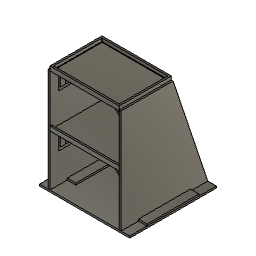
Restaurant Robot Server (v6) (Autodesk Fusion 360 design; units mm, degrees)
Autodesk Fusion 360 part; units mm, degrees
sketch "Sketch1" plane through (0, 0, 0) normal (1, 0, 0) x (0, 1, 0)
  line L0 (0, 0) -> (500, 0)
  line L1 (0, 0) -> (0, 600)
  line L2 (0, 600) -> (300, 600)
  line L3 (300, 600) -> (500, 0)
  dimension "d5" = 600
  constraint coincident L0.start L1.start
  constraint perpendicular L0 L1
  constraint perpendicular L1 L2
  measures "d5" distance of L0.start L1.end
extrude "Extrude1" add sketch "Sketch1" along normal blind 10 makes body 1
move_body "Move1" bodies 1 to x (1, 0, 0) y (0, 1, 0) z (0, 0, 1) at (400, 0, 0)
sketch "Sketch2" plane through (0, 0, 0) normal (1, 0, 0) x (0, 1, 0)
  line L0 (500, 0) -> (0, 0)
  line L1 (0, 0) -> (0, 600)
  line L2 (0, 600) -> (300, 600)
  line L3 (500, 0) -> (300, 600)
  constraint coincident L0.end L1.start
  constraint perpendicular L0 L1
  constraint perpendicular L1 L2
extrude "Extrude2" add sketch "Sketch2" against normal blind 10 separate body makes body 2
move_body "Move2" bodies 2 1 to x (1, 0, 0) y (0, 1, 0) z (0, 0, 1) at (0, 0, 300)
sketch "Sketch3" plane through (0, 0, 300) normal (0, 0, -1) x (1, 0, 0)
  line L0 (0, -500) -> (0, 0)
  line L1 (0, 0) -> (-10, 0)
  line L2 (-10, 0) -> (-10, -500)
  line L3 (-10, -500) -> (0, -500)
  line L4 (-10, -400) -> (0, -400)
  line L5 (0, -400) -> (0, -100)
  line L6 (0, -100) -> (-10, -100)
  line L7 (-10, -100) -> (-10, -400)
  constraint coincident L2 L4.start
  constraint horizontal L4
  constraint vertical L5
  constraint horizontal L6
  constraint vertical L7
  constraint coincident L0 L5.end
extrude "Extrude3" add sketch "Sketch3" along normal blind 50 contours L0 L2 L4 L5 L6 L7 bodies 2
sketch "Sketch4" plane through (0, 0, 300) normal (0, 0, -1) x (1, 0, 0)
  line L0 (400, 0) -> (400, -500)
  line L1 (400, -500) -> (410, -500)
  line L2 (410, -500) -> (410, 0)
  line L3 (410, 0) -> (400, 0)
  line L4 (400, -100) -> (410, -100)
  line L5 (410, -100) -> (410, -400)
  line L6 (410, -400) -> (400, -400)
  line L7 (400, -400) -> (400, -100)
  dimension "d8" = 300
  constraint coincident L0 L4.start
  constraint horizontal L4
  constraint vertical L5
  constraint horizontal L6
  constraint vertical L7
  measures "d8" distance of L4.start L6.end
extrude "Extrude4" add sketch "Sketch4" along normal blind 50 contours L0 L2 L4 L5 L6 L7 bodies 1
sketch "Sketch5" plane through (410, 0, 0) normal (1, 0, 0) x (0, 1, 0)
  line L0 (0, 300) -> (100, 300)
  line L1 (100, 300) -> (100, 250)
  line L2 (100, 250) -> (400, 250)
  line L3 (400, 250) -> (400, 300)
  line L4 (400, 300) -> (500, 300)
  line L5 (500, 300) -> (300, 900)
  line L6 (300, 900) -> (0, 900)
  line L7 (0, 900) -> (0, 300)
  line L8 (100, 300) -> (400, 300)
  line L9 (400, 300) -> (400, 310)
  line L10 (400, 310) -> (100, 310)
  line L11 (100, 310) -> (100, 300)
  constraint horizontal L8
  constraint vertical L9
  constraint horizontal L10
  constraint vertical L11
  constraint coincident L0.end L1.start
extrude "Extrude5" add sketch "Sketch5" along normal blind 50 contours L8 L9 L10 L11 bodies 1
sketch "Sketch6" plane through (400, 0, 0) normal (-1, 0, 0) x (0, -1, 0)
  line L0 (-100, 300) -> (0, 300)
  line L1 (0, 300) -> (0, 900)
  line L2 (0, 900) -> (-300, 900)
  line L3 (-300, 900) -> (-500, 300)
  line L4 (-500, 300) -> (-400, 300)
  line L5 (-400, 300) -> (-400, 250)
  line L6 (-400, 250) -> (-100, 250)
  line L7 (-100, 250) -> (-100, 300)
  line L8 (-400, 310) -> (-100, 310)
  line L9 (-100, 310) -> (-100, 300)
  line L10 (-100, 300) -> (-400, 300)
  line L11 (-400, 300) -> (-400, 310)
  constraint horizontal L8
  constraint vertical L9
  constraint horizontal L10
  constraint vertical L11
  constraint coincident L0.start L7.end
extrude "Extrude6" add sketch "Sketch6" along normal blind 50 contours L8 L9 L10 L11 bodies 1
sketch "Sketch7" plane through (0, 0, 0) normal (1, 0, 0) x (0, 1, 0)
  line L0 (400, 300) -> (500, 300)
  line L1 (500, 300) -> (300, 900)
  line L2 (300, 900) -> (0, 900)
  line L3 (0, 900) -> (0, 300)
  line L4 (0, 300) -> (100, 300)
  line L5 (100, 300) -> (100, 250)
  line L6 (100, 250) -> (400, 250)
  line L7 (400, 250) -> (400, 300)
  line L8 (100, 310) -> (400, 310)
  line L9 (400, 310) -> (400, 300)
  line L10 (400, 300) -> (100, 300)
  line L11 (100, 300) -> (100, 310)
  constraint horizontal L8
  constraint vertical L9
  constraint horizontal L10
  constraint vertical L11
  constraint coincident L0.start L7.end
extrude "Extrude7" add sketch "Sketch7" along normal blind 50 contours L8 L9 L10 L11 bodies 2
sketch "Sketch8" plane through (-10, 0, 0) normal (-1, 0, 0) x (0, -1, 0)
  line L0 (-500, 300) -> (-400, 300)
  line L1 (-400, 300) -> (-400, 250)
  line L2 (-400, 250) -> (-100, 250)
  line L3 (-100, 250) -> (-100, 300)
  line L4 (-100, 300) -> (0, 300)
  line L5 (0, 300) -> (0, 900)
  line L6 (0, 900) -> (-300, 900)
  line L7 (-300, 900) -> (-500, 300)
  line L8 (-400, 300) -> (-100, 300)
  line L9 (-100, 300) -> (-100, 310)
  line L10 (-100, 310) -> (-400, 310)
  line L11 (-400, 310) -> (-400, 300)
  constraint horizontal L8
  constraint vertical L9
  constraint horizontal L10
  constraint vertical L11
  constraint coincident L0.end L1.start
extrude "Extrude8" add sketch "Sketch8" along normal blind 50 contours L8 L9 L10 L11 bodies 2
sketch "Sketch9" plane through (0, 0, 0) normal (0, 0, 1) x (1, 0, 0)
  line L0 (-60, 0) -> (460, 0)
  line L1 (-60, 0) -> (460, 0)
  line L2 (460, 0) -> (460, 500)
  line L3 (460, 500) -> (-60, 500)
  line L4 (-60, 500) -> (-60, 0)
  constraint horizontal L1
  constraint vertical L2
  constraint horizontal L3
  constraint vertical L4
sketch "Sketch18" plane through (0, 0, 0) normal (0, 1, 0) x (1, 0, 0)
  line L0 (0, 0) -> (0, -100)
  line L1 (0, -100) -> (100, -100)
  line L2 (100, -100) -> (0, 0)
  line L3 (0, -100) -> (0, -90)
  line L4 (50, -50) -> (42.9289, -57.0711)
  line L5 (42.9289, -57.0711) -> (75.8579, -90)
  line L6 (42.9289, -57.0711) -> (10, -24.1421)
  line L7 (10, -24.1421) -> (10, -90)
  line L8 (10, -90) -> (75.8579, -90)
  line L9 (75.8579, -90) -> (10, -24.1421)
  dimension "d52" = 10
  constraint coincident L0.start L2.end
  constraint vertical L0
  constraint perpendicular L0 L1
  constraint coincident L0 L3.end
  constraint midpoint L2 L4.start
  constraint perpendicular L4 L5
  constraint perpendicular L4 L6
  measures "d52" distance of L4.start L4.end
extrude "Extrude20" add sketch "Sketch18" along normal blind 30 separate body makes body 3
move_body "Move4" bodies 3 to x (1, 0, 0) y (0, 1, 0) z (0, 0, 1) at (0, 50, 770)
combine "Combine1" operation add target body 3 tool bodies 2
extrude "Extrude21" add sketch "Sketch18" along normal blind 30 separate body makes body 4
move_body "Move5" bodies 4 to x (1, 0, 0) y (0, 1, 0) z (0, 0, 1) at (0, 250, 770)
combine "Combine2" operation add target body 4 tool bodies 3
extrude "Extrude22" add sketch "Sketch18" along normal blind 30 separate body makes body 5
move_body "Move6" bodies 5 to x (1, 0, 0) y (0, 1, 0) z (0, 0, 1) at (0, 50, 470)
extrude "Extrude23" add sketch "Sketch18" along normal blind 30 separate body makes body 6
move_body "Move7" bodies 6 to x (1, 0, 0) y (0, 1, 0) z (0, 0, 1) at (0, 250, 470)
extrude "Extrude24" add sketch "Sketch18" along normal blind 30 separate body makes body 7
move_body "Move8" bodies 7 to x (-1, 0, 0) y (0, -1, 0) z (0, 0, 1) at (0, 0, 0)
move_body "Move9" bodies 7 to x (1, 0, 0) y (0, 1, 0) z (0, 0, 1) at (400, 50, 770)
extrude "Extrude25" add sketch "Sketch18" along normal blind 30 separate body makes body 8
move_body "Move10" bodies 8 to x (-1, 0, 0) y (0, -1, 0) z (0, 0, 1) at (0, 0, 0)
move_body "Move11" bodies 8 to x (1, 0, 0) y (0, 1, 0) z (0, 0, 1) at (400, 250, 770)
extrude "Extrude26" add sketch "Sketch18" along normal blind 30 separate body makes body 9
move_body "Move12" bodies 9 to x (-1, 0, 0) y (0, -1, 0) z (0, 0, 1) at (0, 0, 0)
move_body "Move13" bodies 7 to x (1, 0, 0) y (0, 1, 0) z (0, 0, 1) at (0, 30, 0)
move_body "Move14" bodies 8 to x (1, 0, 0) y (0, 1, 0) z (0, 0, 1) at (0, 30, 0)
move_body "Move15" bodies 9 to x (1, 0, 0) y (0, 1, 0) z (0, 0, 1) at (400, 80, 470)
extrude "Extrude27" add sketch "Sketch18" along normal blind 30 separate body makes body 10
move_body "Move16" bodies 10 to x (-1, 0, 0) y (0, -1, 0) z (0, 0, 1) at (400, 280, 470)
combine "Combine3" operation add target body 7 tool bodies 1 8 9 10
combine "Combine4" operation add target body 6 tool bodies 5 4
sketch "Sketch19" plane through (0, 0, 870) normal (0, 0, 1) x (-1, 0, 0)
  line L0 (-400, -80) -> (-300, -80)
  line L1 (-300, -80) -> (-300, -50)
  line L2 (-300, -50) -> (-400, -50)
  line L3 (-400, -50) -> (-400, -80)
  line L4 (-390, -70) -> (-310, -70)
  line L5 (-310, -70) -> (-310, -60)
  line L6 (-310, -60) -> (-390, -60)
  line L7 (-390, -60) -> (-390, -70)
  line L8 (-390, -270) -> (-310, -270)
  line L9 (-310, -270) -> (-310, -260)
  line L10 (-310, -260) -> (-390, -260)
  line L11 (-390, -260) -> (-390, -270)
  constraint horizontal L4
  constraint vertical L5
  constraint horizontal L6
  constraint vertical L7
  constraint horizontal L8
  constraint vertical L9
  constraint horizontal L10
  constraint vertical L11
extrude "Extrude28" add sketch "Sketch19" along normal blind 20 contours L4 L5 L6 L7 | L8 L9 L10 L11 bodies 7
sketch "Sketch20" plane through (0, 0, 870) normal (0, 0, 1) x (-1, 0, 0)
  line L0 (0, -250) -> (-100, -250)
  line L1 (-100, -250) -> (-100, -280)
  line L2 (-100, -280) -> (0, -280)
  line L3 (0, -280) -> (0, -250)
  line L4 (-90, -60) -> (-10, -60)
  line L5 (-10, -60) -> (-10, -70)
  line L6 (-10, -70) -> (-90, -70)
  line L7 (-90, -70) -> (-90, -60)
  line L8 (-90, -260) -> (-10, -260)
  line L9 (-10, -260) -> (-10, -270)
  line L10 (-10, -270) -> (-90, -270)
  line L11 (-90, -270) -> (-90, -260)
  constraint horizontal L4
  constraint vertical L5
  constraint horizontal L6
  constraint vertical L7
  constraint horizontal L8
  constraint vertical L9
  constraint horizontal L10
  constraint vertical L11
extrude "Extrude29" add sketch "Sketch20" along normal blind 20 contours L4 L5 L6 L7 | L8 L9 L10 L11 bodies 6
sketch "Sketch21" plane through (0, 0, 570) normal (0, 0, 1) x (-1, 0, 0)
  line L0 (-400, -280) -> (-300, -280)
  line L1 (-300, -280) -> (-300, -250)
  line L2 (-300, -250) -> (-400, -250)
  line L3 (-400, -250) -> (-400, -280)
  line L4 (-310, -270) -> (-390, -270)
  line L5 (-390, -270) -> (-390, -260)
  line L6 (-390, -260) -> (-310, -260)
  line L7 (-310, -260) -> (-310, -270)
  line L8 (-310, -70) -> (-390, -70)
  line L9 (-390, -70) -> (-390, -60)
  line L10 (-390, -60) -> (-310, -60)
  line L11 (-310, -60) -> (-310, -70)
  line L12 (-10, -70) -> (-90, -70)
  line L13 (-90, -70) -> (-90, -60)
  line L14 (-90, -60) -> (-10, -60)
  line L15 (-10, -60) -> (-10, -70)
  line L16 (-10, -270) -> (-90, -270)
  line L17 (-90, -270) -> (-90, -260)
  line L18 (-90, -260) -> (-10, -260)
  line L19 (-10, -260) -> (-10, -270)
  constraint horizontal L4
  constraint vertical L5
  constraint horizontal L6
  constraint vertical L7
  constraint horizontal L8
  constraint vertical L9
  constraint horizontal L10
  constraint vertical L11
  constraint horizontal L12
  constraint vertical L13
  constraint horizontal L14
  constraint vertical L15
  constraint horizontal L16
  constraint vertical L17
  constraint horizontal L18
  constraint vertical L19
extrude "Extrude30" add sketch "Sketch21" along normal blind 20 contours L4 L5 L6 L7 | L8 L9 L10 L11 | L12 L13 L14 L15 | L16 L17 L18 L19 bodies 6 7
sketch "Sketch22" plane through (0, 0, 900) normal (0, 0, 1) x (-1, 0, 0)
  line L0 (-400, -300) -> (-400, 0)
  line L1 (-400, 0) -> (-410, 0)
  line L2 (-410, 0) -> (-410, -300)
  line L3 (-410, -300) -> (-400, -300)
  line L4 (-400, 0) -> (0, 0)
  line L5 (0, 0) -> (0, -300)
  line L6 (0, -300) -> (-400, -300)
  line L7 (-400, -300) -> (-400, 0)
  dimension "d75" = 400
  dimension "d76" = 300
  constraint horizontal L4
  constraint vertical L5
  constraint horizontal L6
  constraint vertical L7
  constraint coincident L0.end L1.start
  measures "d75" distance of L0.end L4.end
  measures "d76" distance of L0.end L0.start
sketch "Sketch23" plane through (0, 0, 900) normal (0, 0, 1) x (1, 0, 0)
  line L0 (390, 60) -> (310, 60)
  line L1 (310, 60) -> (310, 70)
  line L2 (310, 70) -> (390, 70)
  line L3 (390, 70) -> (390, 60)
  line L4 (390, 260) -> (310, 260)
  line L5 (310, 260) -> (310, 270)
  line L6 (310, 270) -> (390, 270)
  line L7 (390, 270) -> (390, 260)
  line L8 (90, 260) -> (10, 260)
  line L9 (10, 260) -> (10, 270)
  line L10 (10, 270) -> (90, 270)
  line L11 (90, 270) -> (90, 260)
  line L12 (90, 60) -> (10, 60)
  line L13 (10, 60) -> (10, 70)
  line L14 (10, 70) -> (90, 70)
  line L15 (90, 70) -> (90, 60)
  constraint horizontal L0
  constraint vertical L1
  constraint horizontal L2
  constraint vertical L3
  constraint horizontal L4
  constraint vertical L5
  constraint horizontal L6
  constraint vertical L7
  constraint horizontal L8
  constraint vertical L9
  constraint horizontal L10
  constraint vertical L11
  constraint horizontal L12
  constraint vertical L13
  constraint horizontal L14
  constraint vertical L15
sketch "Sketch24" plane through (0, 0, 900) normal (0, 0, 1) x (-1, 0, 0)
  line L0 (-400, -50) -> (0, -50)
  line L1 (0, -50) -> (0, -80)
  line L2 (0, -80) -> (-400, -80)
  line L3 (-400, -80) -> (-400, -50)
  line L4 (-400, -250) -> (0, -250)
  line L5 (0, -250) -> (0, -280)
  line L6 (0, -280) -> (-400, -280)
  line L7 (-400, -280) -> (-400, -250)
  constraint horizontal L0
  constraint vertical L1
  constraint horizontal L2
  constraint vertical L3
  constraint horizontal L4
  constraint vertical L5
  constraint horizontal L6
  constraint vertical L7
extrude "Extrude1'" add sketch "Sketch24" against normal blind 30 separate body makes body 11 at (266.6667, 50, 890) makes body 12 at (266.6667, 250, 890) in component "Component"
extrude "Extrude2'" cut 1 faces at (266.6667, 260, 900) along direction (0, 0, -1) blind 5 on bodies 12 bodies 12 in component "Component"
extrude "Extrude3'" cut 1 faces at (266.6667, 60, 900) along direction (0, 0, -1) blind 5 on bodies 11 bodies 11 in component "Component"
move_body "Move1'" bodies 12 11 to x (1, 0, 0) y (0, 1, 0) z (0, 0, 1) at (0, 0, 30) in component "Component"
extrude "Extrude4'" cut sketch "Sketch23" along normal blind 20 bodies 11 12 in component "Component"
move_body "Move2'" bodies 11 12 to x (1, 0, 0) y (0, 1, 0) z (0, 0, 1) at (0, 0, -30) in component "Component"
extrude "Extrude1''" add sketch "Sketch22" against normal blind 5 separate body contours L0 L4 L5 L6 L7 makes body 13 in component "Component'"
combine "Combine1'" operation add target body 13 tool bodies 12 11 in component "Component'"
move_body "Move1''" bodies 13 to x (1, 0, 0) y (0, 1, 0) z (0, 0, 1) at (0, 0, 300) in component "Component'"
move_body "Move2''" bodies 13 to x (1, 0, 0) y (0, 1, 0) z (0, 0, 1) at (0, 0, -300) in component "Component'"
move_body "Move3" bodies 13 to x (1, 0, 0) y (0, 1, 0) z (0, 0, 1) at (0, 0, 50) in component "Component'"
move_body "Move4'" bodies 13 to x (1, 0, 0) y (0, 1, 0) z (0, 0, 1) at (0, 0, -50) in component "Component'"
move_body "Move5'" bodies 13 to x (1, 0, 0) y (0, 1, 0) z (0, 0, 1) at (0, 0, 200) in component "Component'"
extrude "Extrude1'''" add sketch "Sketch24" against normal blind 30 separate body makes body 14 at (266.6667, 250, 890) makes body 15 at (266.6667, 50, 890) in component "Component''"
move_body "Move1'''" bodies 14 15 to x (1, 0, 0) y (0, 1, 0) z (0, 0, 1) at (0, 0, 30) in component "Component''"
extrude "Extrude2''" cut sketch "Sketch23" along normal blind 20 bodies 14 15 in component "Component''"
extrude "Extrude3''" cut 2 faces at (266.6667, 260, 930) (266.6667, 60, 930) along direction (0, 0, -1) blind 5 on bodies 14 15 bodies 14 15 in component "Component''"
move_body "Move2'''" bodies 14 15 to x (1, 0, 0) y (0, 1, 0) z (0, 0, 1) at (0, 0, -30) in component "Component''"
sketch "Sketch25" plane through (0, 0, 895) normal (0, 0, 1) x (-1, 0, 0)
  line L0 (-400, -280) -> (0, -280)
  line L1 (0, -280) -> (0, -250)
  line L2 (0, -250) -> (-400, -250)
  line L3 (-400, -250) -> (-400, -280)
  line L4 (-400, 0) -> (0, 0)
  line L5 (0, 0) -> (0, -400)
  line L6 (0, -400) -> (-400, -400)
  line L7 (-400, -400) -> (-400, 0)
  dimension "d93" = 400
  dimension "d94" = 400
  constraint horizontal L4
  constraint vertical L5
  constraint horizontal L6
  constraint vertical L7
  measures "d93" distance of L4.start L4.end
  measures "d94" distance of L4.start L6.end
extrude "Extrude1''''" add sketch "Sketch25" along normal blind 5 separate body makes body 16 in component "Component'''"
combine "Combine1''" operation add target body 15 tool bodies 14 16 in component "Component''"
move_body "Move3'" bodies 15 to x (1, 0, 0) y (0, 1, 0) z (0, 0, 1) at (0, 0, 70) in component "Component''"
move_body "Move6'" bodies 13 to x (1, 0, 0) y (0, 1, 0) z (0, 0, 1) at (0, 0, -200) in component "Component'"
move_body "Move4''" bodies 15 to x (1, 0, 0) y (0, 1, 0) z (0, 0, 1) at (0, 0, -370) in component "Component''"
sketch "Sketch26" plane through (0, 0, 600) normal (0, 0, 1) x (-1, 0, 0)
  line L0 (-400, -400) -> (0, -400)
  line L1 (0, -400) -> (0, 0)
  line L2 (0, 0) -> (-400, 0)
  line L3 (-400, 0) -> (-400, -400)
  line L4 (-400, -400) -> (0, -400)
  line L5 (0, -400) -> (0, -390)
  line L6 (0, -390) -> (-400, -390)
  line L7 (-400, -390) -> (-400, -400)
  dimension "d97" = 10
  constraint horizontal L4
  constraint vertical L5
  constraint horizontal L6
  constraint vertical L7
  constraint coincident L1 L5.end
  constraint coincident L0.start L3.end
  measures "d97" distance of L0.start L6.end
extrude "Extrude31" [suppressed]
extrude "Extrude4''" add sketch "Sketch26" along normal blind 20 contours L0 L1 L3 L4 L5 L6 L7 bodies 15 in component "Component''"
sketch "Sketch27" plane through (0, 0, 0) normal (-1, 0, 0) x (0, -1, 0)
  line L0 (-80, 595) -> (-80, 570)
  line L1 (-80, 570) -> (-50, 570)
  line L2 (-50, 570) -> (-50, 595)
  line L3 (-50, 595) -> (0, 595)
  line L4 (0, 595) -> (0, 600)
  line L5 (0, 600) -> (-390, 600)
  line L6 (-390, 600) -> (-390, 620)
  line L7 (-390, 620) -> (-400, 620)
  line L8 (-400, 620) -> (-400, 595)
  line L9 (-400, 595) -> (-280, 595)
  line L10 (-280, 595) -> (-280, 570)
  line L11 (-280, 570) -> (-250, 570)
  line L12 (-250, 570) -> (-250, 595)
  line L13 (-250, 595) -> (-80, 595)
  line L14 (-400, 620) -> (-400, 600)
  line L15 (-400, 620) -> (-393.333, 620)
  line L16 (-393.333, 620) -> (-400, 600)
  constraint coincident L7.end L8.start
  constraint coincident L8 L14.end
  constraint perpendicular L7 L14
  constraint coincident L7 L15.end
  constraint perpendicular L14 L15
extrude "Extrude5'" cut sketch "Sketch27" against normal blind 400 contours L7 L8 L14 L15 L16 bodies 15 in component "Component''"
fillet "Fillet1" radius 2 1 edges at (200, 390, 600) on bodies 15 in component "Component''"
sketch "Sketch29" plane through (0, 0, 900) normal (0, 0, 1) x (-1, 0, 0)
  line L0 (-400, -300) -> (0, -300)
  line L1 (0, -300) -> (0, 0)
  line L2 (0, 0) -> (-400, 0)
  line L3 (-400, 0) -> (-400, -300)
  line L4 (0, -300) -> (-400, -300)
  line L5 (-400, -300) -> (-400, -290)
  line L6 (-400, -290) -> (0, -290)
  line L7 (0, -290) -> (0, -300)
  line L8 (0, -290) -> (-10, -290)
  line L9 (-10, -290) -> (-10, -10)
  line L10 (-10, -10) -> (0, -10)
  line L11 (0, -10) -> (0, -290)
  line L12 (0, -10) -> (-400, -10)
  line L13 (-400, -10) -> (-400, 0)
  line L14 (-400, 0) -> (0, 0)
  line L15 (0, 0) -> (0, -10)
  line L16 (-400, -10) -> (-390, -10)
  line L17 (-390, -10) -> (-390, -290)
  line L18 (-390, -290) -> (-400, -290)
  line L19 (-400, -290) -> (-400, -10)
  dimension "d108" = 400
  dimension "d109" = 10
  dimension "d114" = 10
  dimension "d115" = 280
  dimension "d116" = 10
  dimension "d117" = 280
  constraint horizontal L4
  constraint vertical L5
  constraint horizontal L6
  constraint vertical L7
  constraint coincident L0.end L1.start
  constraint horizontal L8
  constraint vertical L9
  constraint horizontal L10
  constraint vertical L11
  constraint horizontal L12
  constraint vertical L13
  constraint horizontal L14
  constraint vertical L15
  constraint coincident L2.end L3.start
  constraint horizontal L16
  constraint vertical L17
  constraint horizontal L18
  constraint vertical L19
  measures "d108" distance of L0.end L0.start
  measures "d109" distance of L0.end L6.end
  measures "d114" distance of L6.end L8.end
  measures "d115" distance of L6.end L10.end
  measures "d116" distance of L12.end L16.end
  measures "d117" distance of L12.end L5.end
extrude "Extrude2'''" add sketch "Sketch29" along normal blind 20 contours L0 L1 L3 L4 L5 L6 L7 L8 L18 bodies 13 in component "Component'"
fillet "Fillet1'" radius 2 1 edges at (200, 290, 900) on bodies 13 in component "Component'"
extrude "Extrude3'''" add sketch "Sketch29" along normal blind 20 contours L3 L6 L12 L16 L17 L18 L19 | L1 L6 L8 L9 L10 L11 L12 | L1 L2 L3 L10 L12 L13 L14 L15 L16 bodies 13 in component "Component'"
fillet "Fillet2" radius 2 7 edges at (10, 290, 911) (10, 289.4142, 900.5858) (10, 149, 900) (200, 10, 900) (390, 149, 900) (390, 289.4142, 900.5858) (390, 290, 911) on bodies 13 in component "Component'"
sketch "Sketch30" plane through (0, 0, 600) normal (0, 0, 1) x (-1, 0, 0)
  line L0 (-400, -388) -> (0, -388)
  line L1 (0, -388) -> (0, 0)
  line L2 (0, 0) -> (-400, 0)
  line L3 (-400, 0) -> (-400, -388)
  line L4 (0, -10) -> (-400, -10)
  line L5 (-400, -10) -> (-400, 0)
  line L6 (-400, 0) -> (0, 0)
  line L7 (0, 0) -> (0, -10)
  constraint horizontal L4
  constraint vertical L5
  constraint horizontal L6
  constraint vertical L7
  constraint coincident L2.end L3.start
  constraint coincident L1 L4.start
extrude "Extrude6'" add sketch "Sketch30" along normal blind 20 contours L1 L2 L3 L4 L5 L6 L7 bodies 15 in component "Component''"
fillet "Fillet2'" radius 2 1 edges at (200, 10, 600) on bodies 15 in component "Component''"
sketch "Sketch31" plane through (0, 0, 250) normal (0, 0, -1) x (1, 0, 0)
  line L0 (400, -400) -> (410, -400)
  line L1 (410, -400) -> (410, -100)
  line L2 (410, -100) -> (400, -100)
  line L3 (400, -100) -> (400, -400)
  line L4 (-60, -500) -> (460, -500)
  line L5 (460, -500) -> (460, 0)
  line L6 (460, 0) -> (-60, 0)
  line L7 (-60, 0) -> (-60, -500)
  constraint horizontal L4
  constraint vertical L5
  constraint horizontal L6
  constraint vertical L7
extrude "Extrude1'''''" add sketch "Sketch31" along normal blind 10 separate body makes body 17 in component "Component''''"
move_body "Move1''''" bodies 17 to x (1, 0, 0) y (0, 1, 0) z (0, 0, 1) at (0, 0, -40) in component "Component''''"
sketch "Sketch32" plane through (0, 0, 250) normal (0, 0, -1) x (1, 0, 0)
  line L0 (0, -400) -> (-10, -400)
  line L1 (-10, -400) -> (-10, -100)
  line L2 (-10, -100) -> (0, -100)
  line L3 (0, -100) -> (0, -400)
  dimension "d128" = 10
  dimension "d129" = 300
  constraint horizontal L0
  constraint vertical L1
  constraint horizontal L2
  constraint vertical L3
  measures "d128" distance of L0.start L0.end
  measures "d129" distance of L0.start L2.end
move_body "Move2''''" bodies 17 to x (1, 0, 0) y (0, 1, 0) z (0, 0, 1) at (0, 0, 40) in component "Component''''"
extrude "Extrude2''''" cut sketch "Sketch32" along normal blind 10 bodies 17 in component "Component''''"
move_body "Move3''" bodies 17 to x (1, 0, 0) y (0, 1, 0) z (0, 0, 1) at (0, 0, 50) in component "Component''''"
move_body "Move4'''" bodies 17 to x (1, 0, 0) y (0, 1, 0) z (0, 0, 1) at (0, 0, -200) in component "Component''''"
move_body "Move7'" bodies 13 to x (1, 0, 0) y (0, 1, 0) z (0, 0, 1) at (0, 0, 200) in component "Component'"
move_body "Move5''" bodies 15 to x (1, 0, 0) y (0, 1, 0) z (0, 0, 1) at (0, 0, 700) in component "Component''"
move_body "Move6''" bodies 15 to x (1, 0, 0) y (0, 1, 0) z (0, 0, 1) at (0, 0, -700) in component "Component''"
move_body "Move8'" bodies 13 to x (1, 0, 0) y (0, 1, 0) z (0, 0, 1) at (0, 0, -200) in component "Component'"
move_body "Move5'''" bodies 17 to x (1, 0, 0) y (0, 1, 0) z (0, 0, 1) at (0, 0, 200) in component "Component''''"
component "Component" placed x (1, 0, 0) y (0, 1, 0) z (0, 0, 1) at (0, 0, 0)
component "Component'" placed x (1, 0, 0) y (0, 1, 0) z (0, 0, 1) at (0, 0, 0)
component "Component''" placed x (1, 0, 0) y (0, 1, 0) z (0, 0, 1) at (0, 0, 0)
component "Component'''" placed x (1, 0, 0) y (0, 1, 0) z (0, 0, 1) at (0, 0, 0)
component "Component''''" placed x (1, 0, 0) y (0, 1, 0) z (0, 0, 1) at (0, 0, 0)
